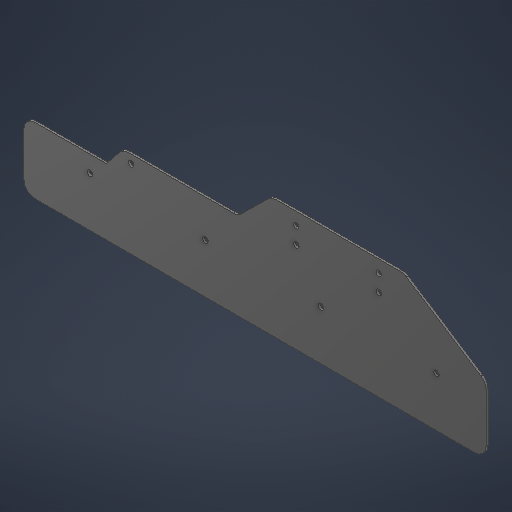
# Autodesk Inventor part: Skirt
Saved by Autodesk Inventor 2025 (Build 290162000, 162)
## iProperties
Created: 2024-12-30
Part Number: Skirt
Material: Generic
Document SubType Name: Modeling
Designer: Juan
Density: 1 g/cm^3
Appearance: Default
Author: Juan
Autodesk Inventor part; units mm, degrees
ref_plane "YZ Plane" through (0, 0, 0) normal (1, 0, 0) x (0, 1, 0)
ref_plane "XZ Plane" through (0, 0, 0) normal (0, 1, 0) x (-1, 0, 0)
ref_plane "XY Plane" through (0, 0, 0) normal (0, 0, 1) x (1, 0, 0)
sketch "Sketch1" plane through (0, 0, 0) normal (0, 0, 1) x (1, 0, 0)
  circle A0 centre (-133.2579, -22.248) radius 2.1844
  circle A1 centre (-101.5079, -0.023) radius 2.2225
  circle A2 centre (-44.3579, -22.248) radius 2.1844
  circle A3 centre (25.4921, 9.502) radius 2.1844
  circle A4 centre (25.4921, 22.202) radius 2.1844
  circle A5 centre (88.9921, 9.502) radius 2.1844
  circle A6 centre (88.9921, 22.202) radius 2.1844
  circle A7 centre (44.5421, -22.248) radius 2.1844
  circle A8 centre (133.4421, -22.248) radius 2.1844
  line L0 (133.4421, -22.248) -> (171.5421, -22.248)
  line L1 (171.5421, -22.248) -> (171.5421, -60.348)
  line L2 (171.5421, -60.348) -> (-184.0579, -60.348)
  line L3 (-184.0579, -60.348) -> (-184.0579, -9.548)
  line L4 (-184.0579, -9.548) -> (-114.2079, -9.548)
  line L5 (-114.2079, -9.548) -> (-114.2079, 6.327)
  line L6 (-19.3781, 6.327) -> (-19.3781, 31.727)
  line L7 (-19.3781, 31.727) -> (6.4421, 31.727)
  line L8 (-19.3781, 6.327) -> (6.4421, 31.727)
  line L9 (6.4421, 31.727) -> (108.0421, 31.727)
  line L10 (108.0421, 31.727) -> (133.1583, 6.1953)
  line L11 (171.5421, -22.248) -> (108.0421, 31.727)
  line L12 (88.9921, 22.202) -> (108.0421, 22.202)
  line L13 (108.0421, 22.202) -> (108.0421, 31.727)
  line L14 (25.4921, 22.202) -> (6.4421, 22.202)
  line L15 (6.4421, 22.202) -> (6.4421, 31.727)
  line L16 (-19.3781, 6.327) -> (-101.5079, 6.327)
  line L17 (-101.5079, 6.327) -> (-114.2079, -9.548)
  line L18 (171.5421, -22.248) -> (171.5421, -9.548)
  line L19 (171.5421, -9.548) -> (108.0421, 31.727)
  line L20 (-114.2079, -9.548) -> (-120.5579, -9.548)
  line L21 (-101.5079, 6.327) -> (-107.8579, 6.327)
  line L22 (-107.8579, 6.327) -> (-120.5579, -9.548)
  point P0 (0, 0)
  dimension "d0" = 38.1
  dimension "d1" = 38.1
  dimension "d2" = 355.6
  dimension "d3" = 50.8
  dimension "d4" = 69.85
  dimension "d5" = 15.875
  dimension "d7" = 25.4
  dimension "d10" = 19.05
  dimension "d11" = 19.05
  dimension "d14" = 12.7
  dimension "d17" = 6.35
  dimension "d18" = 6.35
  constraints: 48 end point, 9 centre point, 7 horizontal, 5 vertical, 4 perpendicular, 1 point on line, 19 other
  measures "d0" distance of L0.start L0.end
  measures "d1" distance of L0.end L1.end
  measures "d2" distance of L1.end L2.end
  measures "d3" distance of L2.end L3.end
  measures "d4" distance of L3.end L4.end
  measures "d5" distance of L4.end L5.end
  measures "d7" distance of L6.start L6.end
  measures "d10" distance of L12.start L12.end
  measures "d11" distance of L14.start L14.end
  measures "d14" distance of L0.end L18.end
  measures "d17" distance of L4.end L20.end
  measures "d18" distance of L16.end L21.end
extrude "Extrusion2" add sketch "Sketch1" along normal blind 1.5875 contours L1 L2 L3 L4 L17 L16 L8 L9 L11 | L22 L5 L4 | L17 L5 L22 L21
extrude "Extrusion3" add sketch "Sketch1" along normal blind 1.5875 contours L11 L19 L18
fillet "Fillet1" radius 8.4667 3 edges at (-107.8579, 6.327, 0.7937) (6.4421, 31.727, 0.7937) (-19.3781, 6.327, 0.7937)
fillet "Fillet2" radius 8.4667 5 edges at (108.0421, 31.727, 0.7937) (171.5421, -9.548, 0.7937) (171.5421, -60.348, 0.7937) (-184.0579, -9.548, 0.7937) (-184.0579, -60.348, 0.7937)
body "Solid2"
